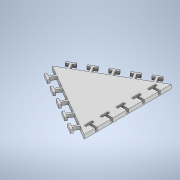
# Autodesk Inventor part: Base2
Saved by Autodesk Inventor 2022.3 (Build 263350000, 350)
## iProperties
Created: 2023-03-28
Part Number: Base2
Material: Generic
Document SubType Name: Modeling
Designer: Manuel Hueso Béjar
Density: 1 g/cm^3
Appearance: Default
Author: Manuel Hueso Béjar
Autodesk Inventor part; units mm, degrees
ref_plane "YZ Plane" through (0, 0, 0) normal (1, 0, 0) x (0, 1, 0)
ref_plane "XZ Plane" through (0, 0, 0) normal (0, 1, 0) x (-1, 0, 0)
ref_plane "XY Plane" through (0, 0, 0) normal (0, 0, 1) x (1, 0, 0)
sketch "Sketch1" plane through (0, 0, 0) normal (0, 1, 0) x (-1, 0, 0)
  circle A0 centre (0, 0) radius 127.0171
  line L0 (127.0171, 0) -> (-63.5085, -110)
  line L1 (-63.5085, -110) -> (-63.5085, 110)
  line L2 (-63.5085, 110) -> (127.0171, 0)
  line L3 (-46.0085, 2.5) -> (-81.0085, 2.5)
  line L4 (-81.0085, 2.5) -> (-81.0085, -2.5)
  line L5 (-81.0085, -2.5) -> (-46.0085, -2.5)
  line L6 (-46.0085, -2.5) -> (-46.0085, 2.5)
  line L7 (-46.0085, 2.5) -> (-81.0085, -2.5) construction
  line L8 (-81.0085, 2.5) -> (-46.0085, -2.5) construction
  line L9 (-48.5085, 10) -> (-43.5085, 10)
  line L10 (-43.5085, 10) -> (-43.5085, -10)
  line L11 (-43.5085, -10) -> (-48.5085, -10)
  line L12 (-48.5085, -10) -> (-48.5085, 10)
  line L13 (-48.5085, 10) -> (-43.5085, -10) construction
  line L14 (-43.5085, 10) -> (-48.5085, -10) construction
  line L15 (-43.5085, 50) -> (-43.5085, 30)
  line L16 (-48.5085, 50) -> (-43.5085, 50)
  line L17 (-48.5085, 30) -> (-48.5085, 50)
  line L18 (-43.5085, 30) -> (-48.5085, 30)
  line L19 (-46.0085, 42.5) -> (-81.0085, 42.5)
  line L20 (-81.0085, 37.5) -> (-46.0085, 37.5)
  line L21 (-43.5085, 90) -> (-43.5085, 70)
  line L22 (-48.5085, 90) -> (-43.5085, 90)
  line L23 (-48.5085, 70) -> (-48.5085, 90)
  line L24 (-43.5085, 70) -> (-48.5085, 70)
  line L25 (-46.0085, 82.5) -> (-81.0085, 82.5)
  line L26 (-81.0085, 77.5) -> (-46.0085, 77.5)
  line L27 (-43.5085, -30) -> (-43.5085, -50)
  line L28 (-48.5085, -30) -> (-43.5085, -30)
  line L29 (-48.5085, -50) -> (-48.5085, -30)
  line L30 (-43.5085, -50) -> (-48.5085, -50)
  line L31 (-46.0085, -37.5) -> (-81.0085, -37.5)
  line L32 (-81.0085, -42.5) -> (-46.0085, -42.5)
  line L33 (-43.5085, 10) -> (-43.5085, -10)
  line L34 (-48.5085, 10) -> (-43.5085, 10)
  line L35 (-48.5085, -10) -> (-48.5085, 10)
  line L36 (-43.5085, -10) -> (-48.5085, -10)
  line L37 (-46.0085, 2.5) -> (-81.0085, 2.5)
  line L38 (-81.0085, -2.5) -> (-46.0085, -2.5)
  line L39 (-43.5085, 50) -> (-43.5085, 30)
  line L40 (-48.5085, 50) -> (-43.5085, 50)
  line L41 (-48.5085, 30) -> (-48.5085, 50)
  line L42 (-43.5085, 30) -> (-48.5085, 30)
  line L43 (-46.0085, 42.5) -> (-81.0085, 42.5)
  line L44 (-81.0085, 37.5) -> (-46.0085, 37.5)
  line L45 (-43.5085, -70) -> (-43.5085, -90)
  line L46 (-48.5085, -70) -> (-43.5085, -70)
  line L47 (-48.5085, -90) -> (-48.5085, -70)
  line L48 (-43.5085, -90) -> (-48.5085, -90)
  line L49 (-46.0085, -77.5) -> (-81.0085, -77.5)
  line L50 (-81.0085, -82.5) -> (-46.0085, -82.5)
  line L51 (-43.5085, -30) -> (-43.5085, -50)
  line L52 (-48.5085, -30) -> (-43.5085, -30)
  line L53 (-48.5085, -50) -> (-48.5085, -30)
  line L54 (-43.5085, -50) -> (-48.5085, -50)
  line L55 (-46.0085, -37.5) -> (-81.0085, -37.5)
  line L56 (-81.0085, -42.5) -> (-46.0085, -42.5)
  line L57 (-43.5085, 10) -> (-43.5085, -10)
  line L58 (-48.5085, 10) -> (-43.5085, 10)
  line L59 (-48.5085, -10) -> (-48.5085, 10)
  line L60 (-43.5085, -10) -> (-48.5085, -10)
  line L61 (-46.0085, 2.5) -> (-81.0085, 2.5)
  line L62 (-81.0085, -2.5) -> (-46.0085, -2.5)
  point P0 (-63.5085, 0)
  point P1 (-46.0085, 0)
  point P2 (-48.5085, 42.5)
  point P3 (-63.5085, 42.5)
  point P4 (-63.5085, 37.5)
  point P5 (-48.5085, 37.5)
  point P6 (-48.5085, -37.5)
  point P7 (-63.5085, -37.5)
  point P8 (-63.5085, -42.5)
  point P9 (-48.5085, -42.5)
  point P10 (-48.5085, 82.5)
  point P11 (-63.5085, 82.5)
  point P12 (-63.5085, 77.5)
  point P13 (-48.5085, 77.5)
  point P14 (-48.5085, -77.5)
  point P15 (-63.5085, -77.5)
  point P16 (-63.5085, -82.5)
  point P17 (-48.5085, -82.5)
  point P18 (-48.5085, -2.5)
  point P19 (-48.5085, 2.5)
  point P20 (-63.5085, 2.5)
  point P21 (-63.5085, -2.5)
  dimension "d1" = 220
  dimension "d2" = 35
  dimension "d3" = 5
  dimension "d4" = 5
  dimension "d5" = 20
  dimension "d8" = 40
  dimension "d11" = 40
  constraints: 126 end point, 6 midpoint, 4 parallel, 2 coincident, 2 horizontal, 2 perpendicular, 2 vertical, 1 horizontal alignment, 121 other
  measures "d1" distance of L0.end L1.end
  measures "d2" distance of L5.end L4.end
  measures "d3" distance of L4.end L3.end
  measures "d4" distance of L10.end L11.end
  measures "d5" distance of L9.end L10.end
  measures "d8" distance of L9.end L15.start
  measures "d11" distance of L9.end L27.start
extrude "Extrusion1" add sketch "Sketch1" along normal blind 10 contours L0 L1 L50 L47 L48 L45 L46 L49 L32 L29 L30 L27 L28 L31 L5 L12 L11 L10 L9 L3 L20 L17 L18 L15 L16 L19 L26 L23 L24 L21 L22 L25 L2 | L25 L23 L26 L1 | L1 L49 L47 L50 | L23 L22 L21 L24 | L47 L46 L45 L48 | L19 L17 L20 L1 | L1 L31 L29 L32 | L17 L16 L15 L18 | L29 L28 L27 L30 | L3 L12 L5 L1 | L12 L9 L10 L11 L5 L6 L3 | L3 L6 L5 L12
extrude "Extrusion2" cut sketch "Sketch1" along normal blind 10 contours L25 L23 L26 L1 | L1 L49 L47 L50 | L23 L22 L21 L24 | L47 L46 L45 L48 | L19 L17 L20 L1 | L1 L31 L29 L32 | L17 L16 L15 L18 | L29 L28 L27 L30 | L3 L12 L5 L1 | L12 L9 L10 L11 L5 L6 L3 | L3 L6 L5 L12
extrude "Extrusion3" add sketch "Sketch1" along normal blind 2.5 contours L25 L23 L26 L1 | L1 L49 L47 L50 | L23 L22 L21 L24 | L47 L46 L45 L48 | L19 L17 L20 L1 | L1 L31 L29 L32 | L17 L16 L15 L18 | L29 L28 L27 L30 | L3 L12 L5 L1 | L12 L9 L10 L11 L5 L6 L3 | L3 L6 L5 L12
sketch "Sketch2" plane through (0, 0, 0) normal (0, -1, 0) x (1, 0, 0)
  line L0 (63.5085, 110) -> (63.5085, -110) projected
  line L1 (-127.0171, 0) -> (63.5085, 110) projected
  line L2 (63.5085, -110) -> (-127.0171, 0) projected
  line L3 (41.5085, 71.8949) -> (41.5085, -71.8949)
  line L4 (41.5085, -71.8949) -> (-83.0171, 0)
  line L5 (-83.0171, 0) -> (41.5085, 71.8949)
  line L6 (36.5085, 63.2346) -> (36.5085, -63.2346)
  line L7 (36.5085, -63.2346) -> (-73.0171, 0)
  line L8 (-73.0171, 0) -> (36.5085, 63.2346)
  point P0 (0, 0)
  dimension "d20" = 22
  dimension "d21" = 5
  constraints: 12 end point, 4 other
  measures "d20" distance between parallel lines of L1 L5
  measures "d21" distance between parallel lines of L5 L8
extrude "Extrusion4" cut sketch "Sketch2" against normal blind 3 contours L3 L4 L5
sketch "Sketch3" plane through (0, 10, 0) normal (0, 1, 0) x (1, 0, 0)
  line L0 (63.5085, 110) -> (-127.0171, 0) projected
  line L1 (-31.7543, 55) -> (-39.2543, 67.9904)
  line L2 (-31.7543, 55) -> (-16.7543, 55) construction
  line L3 (-37.0892, 69.2404) -> (-30.594, 72.9904)
  line L4 (-30.594, 72.9904) -> (-33.094, 77.3205)
  line L5 (-33.094, 77.3205) -> (-50.4145, 67.3205)
  line L6 (-50.4145, 67.3205) -> (-47.9145, 62.9904)
  line L7 (-47.9145, 62.9904) -> (-41.4193, 66.7404)
  line L8 (-31.7543, 55) -> (-33.9193, 53.75)
  line L9 (-33.9193, 53.75) -> (-41.4193, 66.7404)
  line L10 (-33.9193, 53.75) -> (-29.5892, 56.25)
  line L11 (-29.5892, 56.25) -> (-37.0892, 69.2404)
  line L12 (-31.7543, -55) -> (-39.2543, -42.0096) construction
  line L13 (-31.7543, -55) -> (-29.5892, -56.25)
  line L14 (-29.5892, -56.25) -> (-33.9193, -53.75)
  line L15 (-31.7543, -55) -> (-39.2543, -67.9904)
  line L16 (-29.5892, -56.25) -> (-37.0892, -69.2404)
  line L17 (-33.9193, -53.75) -> (-41.4193, -66.7404)
  line L18 (-41.4193, -66.7404) -> (-47.9145, -62.9904)
  line L19 (-30.594, -72.9904) -> (-37.0892, -69.2404)
  line L20 (-47.9145, -62.9904) -> (-50.4145, -67.3205)
  line L21 (-33.094, -77.3205) -> (-30.594, -72.9904)
  line L22 (-50.4145, -67.3205) -> (-33.094, -77.3205)
  line L23 (-85.0555, 47.3205) -> (-82.5555, 42.9904)
  line L24 (-82.5555, 42.9904) -> (-76.0603, 46.7404)
  line L25 (-66.3953, 35) -> (-68.5603, 33.75)
  line L26 (-68.5603, 33.75) -> (-64.2302, 36.25)
  line L27 (-68.5603, 33.75) -> (-76.0603, 46.7404)
  line L28 (-66.3953, 35) -> (-73.8953, 47.9904)
  line L29 (-64.2302, 36.25) -> (-71.7302, 49.2404)
  line L30 (-67.735, 57.3205) -> (-85.0555, 47.3205)
  line L31 (-66.3953, 35) -> (-51.3953, 35) construction
  line L32 (-65.235, 52.9904) -> (-67.735, 57.3205)
  line L33 (-71.7302, 49.2404) -> (-65.235, 52.9904)
  line L34 (-119.6966, 27.3205) -> (-117.1966, 22.9904)
  line L35 (-117.1966, 22.9904) -> (-110.7014, 26.7404)
  line L36 (-101.0363, 15) -> (-103.2014, 13.75)
  line L37 (-103.2014, 13.75) -> (-98.8712, 16.25)
  line L38 (-103.2014, 13.75) -> (-110.7014, 26.7404)
  line L39 (-101.0363, 15) -> (-108.5363, 27.9904)
  line L40 (-98.8712, 16.25) -> (-106.3712, 29.2404)
  line L41 (-102.376, 37.3205) -> (-119.6966, 27.3205)
  line L42 (-101.0363, 15) -> (-86.0363, 15) construction
  line L43 (-99.876, 32.9904) -> (-102.376, 37.3205)
  line L44 (-106.3712, 29.2404) -> (-99.876, 32.9904)
  line L45 (-15.7735, 87.3205) -> (-13.2735, 82.9904)
  line L46 (-13.2735, 82.9904) -> (-6.7783, 86.7404)
  line L47 (2.8868, 75) -> (0.7217, 73.75)
  line L48 (0.7217, 73.75) -> (5.0518, 76.25)
  line L49 (0.7217, 73.75) -> (-6.7783, 86.7404)
  line L50 (2.8868, 75) -> (-4.6132, 87.9904)
  line L51 (5.0518, 76.25) -> (-2.4482, 89.2404)
  line L52 (1.547, 97.3205) -> (-15.7735, 87.3205)
  line L53 (2.8868, 75) -> (17.8868, 75) construction
  line L54 (4.047, 92.9904) -> (1.547, 97.3205)
  line L55 (-2.4482, 89.2404) -> (4.047, 92.9904)
  line L56 (-50.4145, 67.3205) -> (-47.9145, 62.9904)
  line L57 (-47.9145, 62.9904) -> (-41.4193, 66.7404)
  line L58 (-31.7543, 55) -> (-33.9193, 53.75)
  line L59 (-33.9193, 53.75) -> (-29.5892, 56.25)
  line L60 (-33.9193, 53.75) -> (-41.4193, 66.7404)
  line L61 (-31.7543, 55) -> (-39.2543, 67.9904)
  line L62 (-29.5892, 56.25) -> (-37.0892, 69.2404)
  line L63 (-33.094, 77.3205) -> (-50.4145, 67.3205)
  line L64 (-31.7543, 55) -> (-16.7543, 55) construction
  line L65 (-30.594, 72.9904) -> (-33.094, 77.3205)
  line L66 (-37.0892, 69.2404) -> (-30.594, 72.9904)
  line L67 (-85.0555, 47.3205) -> (-82.5555, 42.9904)
  line L68 (-82.5555, 42.9904) -> (-76.0603, 46.7404)
  line L69 (-66.3953, 35) -> (-68.5603, 33.75)
  line L70 (-68.5603, 33.75) -> (-64.2302, 36.25)
  line L71 (-68.5603, 33.75) -> (-76.0603, 46.7404)
  line L72 (-66.3953, 35) -> (-73.8953, 47.9904)
  line L73 (-64.2302, 36.25) -> (-71.7302, 49.2404)
  line L74 (-67.735, 57.3205) -> (-85.0555, 47.3205)
  line L75 (-66.3953, 35) -> (-51.3953, 35) construction
  line L76 (-65.235, 52.9904) -> (-67.735, 57.3205)
  line L77 (-71.7302, 49.2404) -> (-65.235, 52.9904)
  line L78 (18.8675, 107.3205) -> (21.3675, 102.9904)
  line L79 (21.3675, 102.9904) -> (27.8627, 106.7404)
  line L80 (37.5278, 95) -> (35.3627, 93.75)
  line L81 (35.3627, 93.75) -> (39.6928, 96.25)
  line L82 (35.3627, 93.75) -> (27.8627, 106.7404)
  line L83 (37.5278, 95) -> (30.0278, 107.9904)
  line L84 (39.6928, 96.25) -> (32.1928, 109.2404)
  line L85 (36.188, 117.3205) -> (18.8675, 107.3205)
  line L86 (37.5278, 95) -> (52.5278, 95) construction
  line L87 (38.688, 112.9904) -> (36.188, 117.3205)
  line L88 (32.1928, 109.2404) -> (38.688, 112.9904)
  line L89 (-15.7735, 87.3205) -> (-13.2735, 82.9904)
  line L90 (-13.2735, 82.9904) -> (-6.7783, 86.7404)
  line L91 (2.8868, 75) -> (0.7217, 73.75)
  line L92 (0.7217, 73.75) -> (5.0518, 76.25)
  line L93 (0.7217, 73.75) -> (-6.7783, 86.7404)
  line L94 (2.8868, 75) -> (-4.6132, 87.9904)
  line L95 (5.0518, 76.25) -> (-2.4482, 89.2404)
  line L96 (1.547, 97.3205) -> (-15.7735, 87.3205)
  line L97 (2.8868, 75) -> (17.8868, 75) construction
  line L98 (4.047, 92.9904) -> (1.547, 97.3205)
  line L99 (-2.4482, 89.2404) -> (4.047, 92.9904)
  line L100 (-50.4145, 67.3205) -> (-47.9145, 62.9904)
  line L101 (-47.9145, 62.9904) -> (-41.4193, 66.7404)
  line L102 (-31.7543, 55) -> (-33.9193, 53.75)
  line L103 (-33.9193, 53.75) -> (-29.5892, 56.25)
  line L104 (-33.9193, 53.75) -> (-41.4193, 66.7404)
  line L105 (-31.7543, 55) -> (-39.2543, 67.9904)
  line L106 (-29.5892, 56.25) -> (-37.0892, 69.2404)
  line L107 (-33.094, 77.3205) -> (-50.4145, 67.3205)
  line L108 (-31.7543, 55) -> (-16.7543, 55) construction
  line L109 (-30.594, 72.9904) -> (-33.094, 77.3205)
  line L110 (-37.0892, 69.2404) -> (-30.594, 72.9904)
  line L111 (-127.0171, 0) -> (63.5085, -110) projected
  line L112 (63.5085, -110) -> (-127.0171, 0)
  line L113 (2.8868, -75) -> (-4.6132, -62.0096) construction
  line L114 (2.8868, -75) -> (5.0518, -76.25)
  line L115 (5.0518, -76.25) -> (0.7217, -73.75)
  line L116 (0.7217, -73.75) -> (-6.7783, -86.7404)
  line L117 (2.8868, -75) -> (-4.6132, -87.9904)
  line L118 (5.0518, -76.25) -> (-2.4482, -89.2404)
  line L119 (-6.7783, -86.7404) -> (-13.2735, -82.9904)
  line L120 (-13.2735, -82.9904) -> (-15.7735, -87.3205)
  line L121 (4.047, -92.9904) -> (-2.4482, -89.2404)
  line L122 (1.547, -97.3205) -> (4.047, -92.9904)
  line L123 (-15.7735, -87.3205) -> (1.547, -97.3205)
  line L124 (37.5278, -95) -> (30.0278, -82.0096) construction
  line L125 (37.5278, -95) -> (39.6928, -96.25)
  line L126 (39.6928, -96.25) -> (35.3627, -93.75)
  line L127 (35.3627, -93.75) -> (27.8627, -106.7404)
  line L128 (37.5278, -95) -> (30.0278, -107.9904)
  line L129 (39.6928, -96.25) -> (32.1928, -109.2404)
  line L130 (27.8627, -106.7404) -> (21.3675, -102.9904)
  line L131 (21.3675, -102.9904) -> (18.8675, -107.3205)
  line L132 (38.688, -112.9904) -> (32.1928, -109.2404)
  line L133 (36.188, -117.3205) -> (38.688, -112.9904)
  line L134 (18.8675, -107.3205) -> (36.188, -117.3205)
  line L135 (-66.3953, -35) -> (-73.8953, -22.0096) construction
  line L136 (-66.3953, -35) -> (-64.2302, -36.25)
  line L137 (-64.2302, -36.25) -> (-68.5603, -33.75)
  line L138 (-68.5603, -33.75) -> (-76.0603, -46.7404)
  line L139 (-66.3953, -35) -> (-73.8953, -47.9904)
  line L140 (-64.2302, -36.25) -> (-71.7302, -49.2404)
  line L141 (-76.0603, -46.7404) -> (-82.5555, -42.9904)
  line L142 (-82.5555, -42.9904) -> (-85.0555, -47.3205)
  line L143 (-65.235, -52.9904) -> (-71.7302, -49.2404)
  line L144 (-67.735, -57.3205) -> (-65.235, -52.9904)
  line L145 (-85.0555, -47.3205) -> (-67.735, -57.3205)
  line L146 (-31.7543, -55) -> (-39.2543, -42.0096) construction
  line L147 (-31.7543, -55) -> (-29.5892, -56.25)
  line L148 (-29.5892, -56.25) -> (-33.9193, -53.75)
  line L149 (-33.9193, -53.75) -> (-41.4193, -66.7404)
  line L150 (-31.7543, -55) -> (-39.2543, -67.9904)
  line L151 (-29.5892, -56.25) -> (-37.0892, -69.2404)
  line L152 (-41.4193, -66.7404) -> (-47.9145, -62.9904)
  line L153 (-47.9145, -62.9904) -> (-50.4145, -67.3205)
  line L154 (-30.594, -72.9904) -> (-37.0892, -69.2404)
  line L155 (-33.094, -77.3205) -> (-30.594, -72.9904)
  line L156 (-50.4145, -67.3205) -> (-33.094, -77.3205)
  line L157 (2.8868, -75) -> (-4.6132, -62.0096) construction
  line L158 (2.8868, -75) -> (5.0518, -76.25)
  line L159 (5.0518, -76.25) -> (0.7217, -73.75)
  line L160 (0.7217, -73.75) -> (-6.7783, -86.7404)
  line L161 (2.8868, -75) -> (-4.6132, -87.9904)
  line L162 (5.0518, -76.25) -> (-2.4482, -89.2404)
  line L163 (-6.7783, -86.7404) -> (-13.2735, -82.9904)
  line L164 (-13.2735, -82.9904) -> (-15.7735, -87.3205)
  line L165 (4.047, -92.9904) -> (-2.4482, -89.2404)
  line L166 (1.547, -97.3205) -> (4.047, -92.9904)
  line L167 (-15.7735, -87.3205) -> (1.547, -97.3205)
  line L168 (-101.0363, -15) -> (-108.5363, -2.0096) construction
  line L169 (-101.0363, -15) -> (-98.8712, -16.25)
  line L170 (-98.8712, -16.25) -> (-103.2014, -13.75)
  line L171 (-103.2014, -13.75) -> (-110.7014, -26.7404)
  line L172 (-101.0363, -15) -> (-108.5363, -27.9904)
  line L173 (-98.8712, -16.25) -> (-106.3712, -29.2404)
  line L174 (-110.7014, -26.7404) -> (-117.1966, -22.9904)
  line L175 (-117.1966, -22.9904) -> (-119.6966, -27.3205)
  line L176 (-99.876, -32.9904) -> (-106.3712, -29.2404)
  line L177 (-102.376, -37.3205) -> (-99.876, -32.9904)
  line L178 (-119.6966, -27.3205) -> (-102.376, -37.3205)
  line L179 (-66.3953, -35) -> (-73.8953, -22.0096) construction
  line L180 (-66.3953, -35) -> (-64.2302, -36.25)
  line L181 (-64.2302, -36.25) -> (-68.5603, -33.75)
  line L182 (-68.5603, -33.75) -> (-76.0603, -46.7404)
  line L183 (-66.3953, -35) -> (-73.8953, -47.9904)
  line L184 (-64.2302, -36.25) -> (-71.7302, -49.2404)
  line L185 (-76.0603, -46.7404) -> (-82.5555, -42.9904)
  line L186 (-82.5555, -42.9904) -> (-85.0555, -47.3205)
  line L187 (-65.235, -52.9904) -> (-71.7302, -49.2404)
  line L188 (-67.735, -57.3205) -> (-65.235, -52.9904)
  line L189 (-85.0555, -47.3205) -> (-67.735, -57.3205)
  line L190 (-31.7543, -55) -> (-39.2543, -42.0096) construction
  line L191 (-31.7543, -55) -> (-29.5892, -56.25)
  line L192 (-29.5892, -56.25) -> (-33.9193, -53.75)
  line L193 (-33.9193, -53.75) -> (-41.4193, -66.7404)
  line L194 (-31.7543, -55) -> (-39.2543, -67.9904)
  line L195 (-29.5892, -56.25) -> (-37.0892, -69.2404)
  line L196 (-41.4193, -66.7404) -> (-47.9145, -62.9904)
  line L197 (-47.9145, -62.9904) -> (-50.4145, -67.3205)
  line L198 (-30.594, -72.9904) -> (-37.0892, -69.2404)
  line L199 (-33.094, -77.3205) -> (-30.594, -72.9904)
  line L200 (-50.4145, -67.3205) -> (-33.094, -77.3205)
  point P0 (0, 0)
  dimension "d24" = 15
  dimension "d25" = 120
  dimension "d26" = 10
  dimension "d27" = 5
  dimension "d28" = 20
  dimension "d29" = 90
  dimension "d30" = 5
  dimension "d31" = 2.5
  dimension "d32" = 5
  dimension "d35" = 120
  dimension "d39" = 40
  dimension "d42" = 40
  dimension "d47" = 40
  dimension "d50" = 40
  constraints: 398 end point, 6 perpendicular, 2 point on line, 1 collinear, 1 equal length, 1 horizontal, 1 midpoint, 379 other
  measures "d24" distance of L1.start L1.end
  measures "d25" angle of L2 L1
  measures "d26" distance of L1.end L3.end
  measures "d27" distance of L3.end L4.end
  measures "d28" distance of L4.end L5.end
  measures "d29" angle of L5 L4
  measures "d30" distance of L5.end L6.end
  measures "d31" distance of L1.start L8.end
  measures "d32" distance of L8.end L10.end
  measures "d39" distance of L6.end L23.end
  measures "d42" distance of L6.end L45.end
  measures "d47" distance of L12.end L113.end
  measures "d50" distance of L12.end L135.end
extrude "Extrusion5" add sketch "Sketch3" against normal blind 7.5
body "Solid1"
